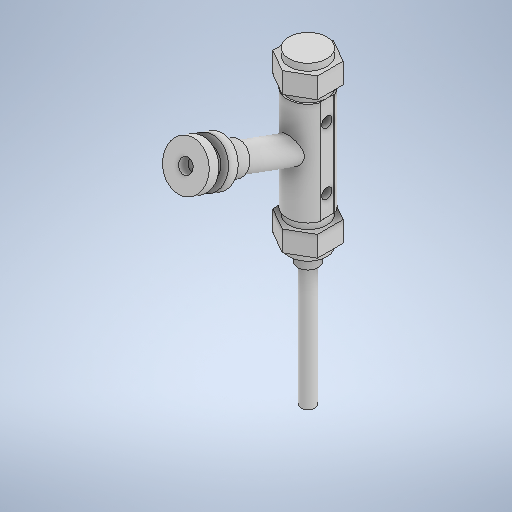
# Autodesk Inventor part: 142
Saved by Autodesk Inventor 2025.1 (Build 291241000, 241)
## iProperties
Created: 2024-08-02
Part Number: 142
Material: Generisch
Document SubType Name: Modeling
Designer: ffogue
Density: 1 g/cm^3
Appearance: Vorgabe
Author: ffogue
Autodesk Inventor part; units mm, degrees
sketch "Skizze1" plane through (0, 0, 0) normal (0, 0, 1) x (1, 0, 0)
  circle A0 centre (0, 0) radius 6
  dimension "d10" = 12
  constraints: 1 centre point, 1 coincident
  measures "d10" diameter of A0
extrude "Extrusion1" add sketch "Skizze1" along normal mid plane 30
ref_plane "Arbeitsebene1" through (0, 0, 0) normal (0, 0, 1) x (1, 0, 0)
sketch "Skizze2" plane through (0, 0, 0) normal (0, 0, 1) x (1, 0, 0)
  circle A0 centre (0, 0) radius 5.5
  dimension "d4" = 11
  constraints: 1 centre point, 1 coincident
  measures "d4" diameter of A0
extrude "Extrusion2" add sketch "Skizze2" along normal mid plane 50
ref_plane "Arbeitsebene2" through (0, 0, -17) normal (0, 0, -1) x (-1, 0, 0)
sketch "Skizze4" plane through (0, 0, -17) normal (0, 0, -1) x (-1, 0, 0)
  circle A0 centre (0, 0) radius 5.5 projected
  line L0 (0, 7.5) -> (6.4952, 3.75)
  line L1 (6.4952, 3.75) -> (6.4952, -3.75)
  line L2 (6.4952, -3.75) -> (0, -7.5)
  line L3 (0, -7.5) -> (-6.4952, -3.75)
  line L4 (-6.4952, -3.75) -> (-6.4952, 3.75)
  line L5 (-6.4952, 3.75) -> (0, 7.5)
  dimension "d11" = 15
  constraints: 12 end point, 1 coincident, 1 vertical alignment, 13 other
  measures "d11" distance of L2.end L0.start
extrude "Extrusion4" add sketch "Skizze4" along normal blind 6
mirror "Spiegeln1" about plane through (0, 0, 0) normal (0, 0, 1) of "Extrusion4"
sketch "Skizze6" plane through (0, 0, -15) normal (0, 0, -1) x (-1, 0, 0)
  circle A0 centre (0, 0) radius 6 projected
  line L0 (5.6569, -2) -> (5.5, -2)
  line L1 (5.5, -2) -> (5.5, 2)
  line L2 (6.4952, -3.75) -> (6.4952, 3.75) projected
  line L3 (5.5, 2) -> (5.6569, 2)
  point P0 (5.5, 0)
  dimension "d16" = 0.5
  dimension "d17" = 4
  constraints: 6 end point, 2 point on circle, 1 horizontal, 1 horizontal alignment, 1 midpoint, 1 parallel, 1 perpendicular
  measures "d16" distance edge to line of A0 L1
  measures "d17" distance between parallel lines of L3 L0
extrude "Extrusion5" cut sketch "Skizze6" against normal up to surface (30 mm away) contours A0 L0 L1 L3 picked at (5.6538, -0.2261)
sketch "Skizze7" plane through (-5.5, 0, -15) normal (-1, 0, 0) x (0, 0, 1)
  point P0 (15, 0)
  point P1 (6, 0)
  point P2 (24, 0)
  dimension "d27" = 9
  dimension "d28" = 18
  constraints: 2 horizontal alignment
  measures "d27" distance of point (15, 0) point (6, 0)
  measures "d28" distance of point (6, 0) point (24, 0)
hole "Bohrung1" at (-5.5, 0, -9) at (-5.5, 0, 9) direction (1, 0, 0) diameter 3 end through all
mirror "Spiegeln2" about plane through (0, 0, 0) normal (1, 0, 0) of "Extrusion5"
ref_plane "Work Plane6" through (0, 0, 0) normal (0, 1, 0) x (-1, 0, 0)
sketch "Sketch15" plane through (0, 0, -25) normal (0, 0, -1) x (-1, 0, 0)
  circle A0 centre (0, 0) radius 3
  dimension "d68" = 6
  constraints: 1 centre point, 1 coincident
  measures "d68" diameter of A0
extrude "Extrusion6" add sketch "Sketch15" along normal blind 4
sketch "Sketch16" plane through (0, 0, -29) normal (0, 0, -1) x (-1, 0, 0)
  point P0 (0, 0)
  point P1 (0.1152, 0.0612)
hole "Hole2" at (-0.1152, 0.0612, -29) direction (0, 0, 1) diameter 4 depth 10
sketch "Sketch17" plane through (-0.1152, 0.0612, -19) normal (0, 0, -1) x (-1, 0, 0)
  circle A0 centre (-0.1152, -0.0612) radius 2
  dimension "d78" = 4
  constraints: 1 centre point, 1 coincident
  measures "d78" diameter of A0
extrude "Extrusion7" add sketch "Sketch17" along normal blind 46 separate body
shell "Shell1" thickness 0.25 removed faces 1 at (-0.6473, -0.1595, -65) bodies 2
ref_plane "Work Plane16" through (0, 0, 0) normal (1, 0, 0) x (0, 1, 0)
sketch "Sketch21" plane through (0, 0, 0) normal (1, 0, 0) x (0, 1, 0)
  line L0 (57.9231, -21.0823) -> (-57.9231, 21.0823) construction
  circle A0 centre (0, 9) radius 1.5 projected
  circle A1 centre (0, -9) radius 1.5 projected
  line L1 (-7.5, -23) -> (-7.5, -17) projected
  line L2 (-7.5, -17) -> (-5.5, -17) projected
  line L3 (-5.5, -17) -> (-5.5, -15) projected
  line L4 (-5.5, -15) -> (-6, -15) projected
  line L5 (-6, -15) -> (-6, 15) projected
  line L6 (-6, 15) -> (-5.5, 15) projected
  line L7 (-5.5, 15) -> (-5.5, 17) projected
  line L8 (-5.5, 17) -> (-7.5, 17) projected
  line L9 (-7.5, 17) -> (-7.5, 23) projected
  line L10 (-7.5, 23) -> (-5.5, 23) projected
  line L11 (-5.5, 23) -> (-5.5, 25) projected
  line L12 (-5.5, 25) -> (5.5, 25) projected
  line L13 (5.5, 25) -> (5.5, 23) projected
  line L14 (5.5, 23) -> (7.5, 23) projected
  line L15 (7.5, 23) -> (7.5, 17) projected
  line L16 (7.5, 17) -> (5.5, 17) projected
  line L17 (5.5, 17) -> (5.5, 15) projected
  line L18 (5.5, 15) -> (6, 15) projected
  line L19 (6, 15) -> (6, -15) projected
  line L20 (6, -15) -> (5.5, -15) projected
  line L21 (5.5, -15) -> (5.5, -17) projected
  line L22 (5.5, -17) -> (7.5, -17) projected
  line L23 (7.5, -17) -> (7.5, -23) projected
  line L24 (7.5, -23) -> (5.5, -23) projected
  line L25 (5.5, -23) -> (5.5, -25) projected
  line L26 (5.5, -25) -> (3, -25) projected
  line L27 (3, -25) -> (3, -29) projected
  line L28 (3, -29) -> (2.0579, -29) projected
  line L29 (2.0579, -29) -> (2.0579, -19) projected
  line L30 (2.0579, -19) -> (-1.9355, -19) projected
  line L31 (-1.9355, -19) -> (-1.9355, -29) projected
  line L32 (-1.9355, -29) -> (-3, -29) projected
  line L33 (-3, -29) -> (-3, -25) projected
  line L34 (-3, -25) -> (-5.5, -25) projected
  line L35 (-5.5, -25) -> (-5.5, -23) projected
  line L36 (-5.5, -23) -> (-7.5, -23) projected
  line L37 (-2, -65) -> (-2, -19) projected
  line L38 (-2, -19) -> (2, -19) projected
  line L39 (2, -19) -> (2, -65) projected
  line L40 (2, -65) -> (1.75, -65) projected
  line L41 (1.75, -65) -> (1.75, -19.25) projected
  line L42 (1.75, -19.25) -> (-1.75, -19.25) projected
  line L43 (-1.75, -19.25) -> (-1.75, -65) projected
  line L44 (-1.75, -65) -> (-2, -65) projected
  line L45 (0, 0) -> (-57.9231, 21.0823)
  point P0 (0, 0)
  point P1 (0, 0)
  point P2 (-28.9615, 10.5411)
  point P3 (-21.5049, 7.8272)
  point P4 (-6, 2.1838)
  dimension "d97" = 70
  dimension "d104" = 16.5
  constraints: 4 end point, 3 midpoint, 3 point on line, 1 coincident, 1 collinear
  measures "d97" angle of L0 L5
  measures "d104" distance of point (-6, 2.184) point (-21.505, 7.827)
ref_plane "Work Plane17" through (0, 57.9231, -21.0823) normal (0, 0, 1) x (1, 0, 0)
sketch "Sketch22" plane through (0, 57.9231, -21.0823) normal (0, 0, 1) x (1, 0, 0)
  line L0 (12.8014, 0) -> (-12.8014, 0) construction
  circle A0 centre (-0.1152, -57.8619) radius 2 projected
  line L1 (0, -50.4231) -> (6.4952, -54.1731) projected
  line L2 (6.4952, -54.1731) -> (6.4952, -61.6731) projected
  line L3 (6.4952, -61.6731) -> (0, -65.4231) projected
  line L4 (0, -65.4231) -> (-6.4952, -61.6731) projected
  line L5 (-6.4952, -61.6731) -> (-6.4952, -54.1731) projected
  line L6 (-6.4952, -54.1731) -> (0, -50.4231) projected
  circle A1 centre (0, -57.9231) radius 1.75 projected
  circle A2 centre (0, -57.9231) radius 2 projected
  point P0 (0, 0)
  point P1 (0, 0)
  constraints: 2 end point, 1 coincident, 1 horizontal, 1 midpoint
ref_plane "Work Plane18" through (12.8014, 57.9231, -21.0823) normal (0, 0.3420201, 0.9396926) x (-1, 0, 0)
ref_plane "Work Plane19" through (0, -57.9231, 21.0823) normal (0, -1, 0) x (1, 0, 0)
ref_plane "Work Plane21" through (0, -21.5049, 7.8272) normal (0, -0.9396926, 0.3420201) x (1, 0, 0)
sketch "Sketch25" plane through (0, -21.5049, 7.8272) normal (0, -0.9396926, 0.3420201) x (1, 0, 0)
  circle A0 centre (0, 0) radius 4.3079
  circle A1 centre (0, 0) radius 3.6661
  circle A2 centre (0, 0) radius 6.4173
  point P0 (0, 0)
  constraints: 3 centre point, 3 coincident
ref_plane "Work Plane24" through (0, -32.7812, 11.9314) normal (0, -0.9396926, 0.3420201) x (1, 0, 0)
ref_plane "Work Plane23" through (0, -29.9622, 10.9053) normal (0, -0.9396926, 0.3420201) x (1, 0, 0)
extrude "Extrusion9" add sketch "Sketch25" against normal up to surface separate body contours A1 round surface about axis through (0, 0, 0) along (0, 0, 1) radius 6 far side no
extrude "Extrusion14" add sketch "Sketch25" along normal blind 6 separate body contours A0 | A1
extrude "Extrusion15" add sketch "Sketch25" along normal blind 3 from surface at 6 separate body contours A0 | A1 | A2
extrude "Extrusion16" add sketch "Sketch25" along normal blind 3 from surface at 9 separate body contours A0 | A1
extrude "Extrusion17" add sketch "Sketch25" along normal blind 3 from surface at 12 separate body contours A0 | A1 | A2
sketch "Sketch26" plane through (0, -35.6003, 12.9575) normal (0, -0.9396926, 0.3420201) x (1, 0, 0)
  circle A0 centre (0, 0) radius 6.4173 projected
  point P0 (0, 0)
  point P1 (0, 0)
  constraints: 1 coincident
hole "Hole3" at (0, -35.6003, 12.9575) direction (0, 0.9396926, -0.3420201) diameter 4 end up to surface bodies 7
sketch "Sketch28" plane through (-5.5, 0, -15) normal (-1, 0, 0) x (0, 0, 1)
  line L0 (30, 2) -> (30, 0) projected
  line L1 (0, 2) -> (30, 2) projected
  line L2 (30, -2) -> (0, -2) projected
  line L3 (30, 0) -> (30, -2) projected
  line L4 (0, -2) -> (0, 0) projected
  line L5 (0, 0) -> (0, 2) projected
  circle A0 centre (24, 0) radius 1.5 projected
  circle A1 centre (6, 0) radius 1.5 projected
  point P0 (15, 0)
sketch "Sketch24" plane through (0, -15.3142, 5.5739) normal (0, -0.9396926, 0.3420201) x (1, 0, 0)
  circle A0 centre (0, 0) radius 5.5
  point P0 (0, 0)
  dimension "d101" = 11
  constraints: 1 centre point, 1 coincident
  measures "d101" diameter of A0
sketch "Sketch23" plane through (0, -57.9231, 21.0823) normal (0, -1, 0) x (1, 0, 0)
  circle A0 centre (0, 0) radius 5.5
  point P0 (0, -21.0823)
  dimension "d98" = 11
  dimension "d85" = 70
  dimension "d86" = 18
  dimension "d87" = 12
  dimension "d88" = 16.2
  dimension "d89" = 18
  dimension "d92" = 2
  dimension "d94" = 8.5
  constraints: 12 end point, 2 parallel, 2 perpendicular, 2 point on circle, 2 point on line, 1 centre point, 1 tangent
ref_plane "Work Plane22" through (0, -27.1431, 9.8793) normal (0, -0.9396926, 0.3420201) x (1, 0, 0)
body "Solid3"
body "Solid4"
body "Solid5"
body "Solid6"
body "Solid7"
body "Solid8"
body "Solid9"
body "Solid10"
body "Solid11"
body "Solid12"
body "Solid13"
body "Srf1"
